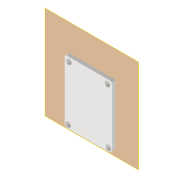
# Autodesk Inventor part: 00_ESP32_XIAO_Adapter_lid
Saved by Autodesk Inventor 2022 (Build 260153000, 153)
## iProperties
Created: 2023-04-27
Part Number: 00_ESP32_XIAO_Adapter_lid
Material: Generisch
Document SubType Name: Modeling
Designer: diederichbenedict
Density: 1 g/cm^3
Appearance: Vorgabe
Author: diederichbenedict
Autodesk Inventor part; units mm, degrees
ref_plane "YZ Plane" through (0, 0, 0) normal (1, 0, 0) x (0, 1, 0)
ref_plane "XZ Plane" through (0, 0, 0) normal (0, 1, 0) x (-1, 0, 0)
ref_plane "XY Plane" through (0, 0, 0) normal (0, 0, 1) x (1, 0, 0)
ref_plane "Arbeitsebene1" through (0, 0, 0) normal (0, 0, 1) x (1, 0, 0)
sketch "Skizze1" plane through (0, 0, 0) normal (0, 0, 1) x (1, 0, 0)
  line L0 (14.5712, 11.3758) -> (14.5712, 4.0068) projected
  line L1 (13.3638, -15.5) -> (13.3638, 1.7) projected
  arc A0 (14.5712, 4.0068) -> (13.3638, 1.7) centre (16.1712, 1.7) ccw projected
  line L2 (10.5793, 11.3758) -> (14.5712, 11.3758) projected
  line L3 (36.5793, 10.3758) -> (36.5793, -24.4) projected
  arc A1 (36.5793, 10.3758) -> (35.5793, 11.3758) centre (35.5793, 10.3758) ccw projected
  line L4 (9.5793, -24.4) -> (9.5793, 10.3758) projected
  line L5 (36.5793, -24.4) -> (9.5793, -24.4) projected
  line L6 (31.5712, 11.3758) -> (35.5793, 11.3758) projected
  line L7 (31.5712, 4.0068) -> (31.5712, 11.3758) projected
  arc A2 (10.5793, 11.3758) -> (9.5793, 10.3758) centre (10.5793, 10.3758) ccw projected
  line L8 (14.5712, 11.3758) -> (31.5712, 11.3758)
  line L9 (9.5793, -24.4) -> (9.5793, 10.3758) projected
  line L10 (36.5793, -24.4) -> (9.5793, -24.4) projected
  line L11 (36.5793, 10.3758) -> (36.5793, -24.4) projected
  circle A3 centre (11.5793, -22.4) radius 1.4 projected
  circle A4 centre (34.0793, 8.8758) radius 1.4 projected
  circle A5 centre (34.5793, -22.4) radius 1.4 projected
  circle A6 centre (12.0793, 8.8758) radius 1.4 projected
  arc A7 (32.7786, 1.7) -> (31.5712, 4.0068) centre (29.9712, 1.7) ccw projected
  line L12 (32.7786, 1.7) -> (32.7786, -15.5) projected
  arc A8 (29.9712, -18.3074) -> (32.7786, -15.5) centre (29.9712, -15.5) ccw projected
  line L13 (29.9712, -18.3074) -> (16.1712, -18.3074) projected
  arc A9 (13.3638, -15.5) -> (16.1712, -18.3074) centre (16.1712, -15.5) ccw projected
  constraints: 2 end point, 1 horizontal
extrude "Extrusion1" add sketch "Skizze1" along normal blind 2 contours L8 L7 A7 L12 A8 L13 A9 L1 A0 L0 | L0 A0 L1 A9 L13 A8 L12 A7 L7 L6 A1 L3 L5 L4 A2 L2 | A3 | A4 | A5 | A6
ref_plane "Arbeitsebene2" through (0, 0, 0) normal (0, 0, 1) x (1, 0, 0)
sketch "Skizze2" plane through (0, 0, 2) normal (0, 0, 1) x (1, 0, 0)
  arc A0 (8.0712, 19) -> (4.0712, 15) centre (8.0712, 15) ccw projected
  line L0 (4.0712, 15) -> (4.0712, -15) projected
  arc A1 (4.0712, -15) -> (8.0712, -19) centre (8.0712, -15) ccw projected
  line L1 (8.0712, -19) -> (38.0712, -19) projected
  arc A2 (38.0712, -19) -> (42.0712, -15) centre (38.0712, -15) ccw projected
  line L2 (42.0712, -15) -> (42.0712, 15) projected
  arc A3 (42.0712, 15) -> (38.0712, 19) centre (38.0712, 15) ccw projected
  line L3 (38.0712, 19) -> (8.0712, 19) projected
  circle A4 centre (8.0712, 15) radius 1.4 projected
  circle A5 centre (38.0712, 15) radius 1.4 projected
  circle A6 centre (38.0712, -15) radius 1.4 projected
  circle A7 centre (8.0712, -15) radius 1.4 projected
  point P0 (0, 0)
hole "Bohrung1" at (8.0712, 15, 2) at (8.0712, -15, 2) at (38.0712, -15, 2) at (38.0712, 15, 2) direction (0, 0, -1) diameter 3.2 end through all
fillet "Rundung1" radius 2 2 edges at (9.5793, -24.4, 1) (36.5793, -24.4, 1)
sketch "Skizze3" plane through (0, 0, 2) normal (0, 0, 1) x (1, 0, 0)
  arc A0 (34.5793, -24.4) -> (36.5793, -22.4) centre (34.5793, -22.4) ccw projected
  line L0 (36.5793, -22.4) -> (36.5793, -15.5783) projected
  arc A1 (36.5793, -14.4217) -> (36.5793, -15.5783) centre (38.0712, -15) ccw projected
  line L1 (36.5793, -14.4217) -> (36.5793, 10.3758) projected
  arc A2 (36.5793, 10.3758) -> (35.5793, 11.3758) centre (35.5793, 10.3758) ccw projected
  line L2 (35.5793, 11.3758) -> (10.5793, 11.3758) projected
  arc A3 (10.5793, 11.3758) -> (9.5793, 10.3758) centre (10.5793, 10.3758) ccw projected
  line L3 (9.5793, 10.3758) -> (9.5793, -14.4657) projected
  arc A4 (9.5793, -15.5343) -> (9.5793, -14.4657) centre (8.0712, -15) ccw projected
  line L4 (9.5793, -15.5343) -> (9.5793, -22.4) projected
  arc A5 (9.5793, -22.4) -> (11.5793, -24.4) centre (11.5793, -22.4) ccw projected
  line L5 (11.5793, -24.4) -> (34.5793, -24.4) projected
  line L6 (34.0793, 8.8758) -> (34.0793, -14.0645)
  arc A6 (34.0793, -14.0645) -> (34.0793, -15.9355) centre (38.0712, -15) ccw
  line L7 (34.0793, -15.9355) -> (34.0793, -21.9)
  line L8 (34.0793, -21.9) -> (12.0793, -21.9)
  line L9 (12.0793, -21.9) -> (12.0793, -15.8629)
  arc A7 (12.0793, -15.8629) -> (12.0793, -14.1371) centre (8.0712, -15) ccw
  line L10 (12.0793, -14.1371) -> (12.0793, 8.8758)
  line L11 (12.0793, 8.8758) -> (34.0793, 8.8758)
  point P0 (0, 0)
  dimension "d13" = 2.5
  constraints: 12 end point, 4 point on circle, 2 centre point, 7 other
  measures "d13" distance between parallel lines of L1 L6
hole "Bohrung2" at (34.5793, -22.4, 2) at (11.5793, -22.4, 2) at (12.0793, 8.8758, 2) at (34.0793, 8.8758, 2) direction (0, 0, -1) diameter 3.2 end through all
